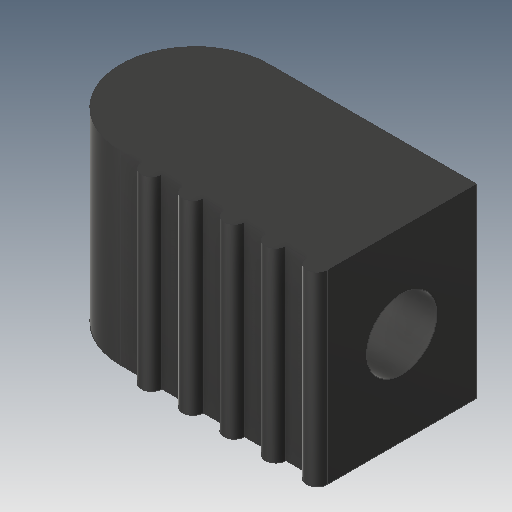
# Autodesk Inventor part: XY_Tensioner
Saved by Autodesk Inventor 2019 (Build 230136000, 136)
## iProperties
Created: 2018-10-20
Part Number: XY_Tensioner
Material: ABS Plastic
Document SubType Name: Modeling
Designer: Ax
Density: 1.06 g/cm^3
Appearance: Smooth - Black
Mass: 0.861327 g
Surface Area: 6.03641 cm^2
Volume: 0.812572 cm^3
Author: Ax
Autodesk Inventor part; units mm, degrees
ref_plane "YZ Plane" through (0, 0, 0) normal (1, 0, 0) x (0, 1, 0)
ref_plane "XZ Plane" through (0, 0, 0) normal (0, 1, 0) x (-1, 0, 0)
ref_plane "XY Plane" through (0, 0, 0) normal (0, 0, 1) x (1, 0, 0)
sketch "Sketch1" plane through (0, 0, 0) normal (0, 1, 0) x (-1, 0, 0)
  arc A0 (0, -3.6) -> (0, 3.6) centre (0, 0) ccw
  line L0 (0, 3.6) -> (-10, 3.6)
  line L1 (-10, 3.6) -> (-10, -3.6)
  line L2 (-10, -3.6) -> (0, -3.6)
  line L3 (0, 3.6) -> (0, -3.6)
  dimension "d0" = 10
  dimension "d1" = 7.2
  constraints: 8 end point, 2 horizontal, 2 point on circle, 1 centre point, 1 coincident, 1 midpoint, 1 perpendicular, 1 vertical
  measures "d0" distance of L0.start L0.end
  measures "d1" distance of L0.end L1.end
extrude "Extrusion1" add sketch "Sketch1" along normal blind 9
sketch "Sketch2" plane through (0, 9, 0) normal (0, 1, 0) x (1, 0, 0)
  line L0 (9, -3.6) -> (10, -3.6)
  arc A0 (9, -3.6) -> (10, -3.6) centre (9.5, -3.6) ccw
  point P0 (0, 0)
  dimension "d4" = 1
  constraints: 2 end point, 2 point on circle, 1 centre point, 1 coincident, 1 horizontal, 1 midpoint
  measures "d4" distance of L0.start L0.end
extrude "Extrusion2" add sketch "Sketch2" against normal blind 9
pattern_linear "Rectangular Pattern1" count 5 spacing 2 along (-1, 0, 0) of "Extrusion2"
sketch "Sketch3" plane through (10, 0, -3.6) normal (1, 0, 0) x (0, 0, -1)
  line L0 (-3.6, 0) -> (-3.6, 9)
  line L1 (0, 9) -> (-7.2, 9) projected
  circle A0 centre (-3.6, 4.5) radius 1.7
  dimension "d10" = 3.4
  constraints: 2 end point, 2 midpoint, 1 centre point
  measures "d10" diameter of A0
extrude "Extrusion3" cut sketch "Sketch3" against normal blind 4
body "Solid1"
